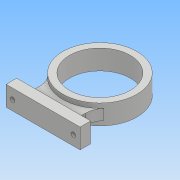
# Autodesk Inventor part: 15528 - 40mm - 1 0.25inch Universal Plastic Pipe Clip c-w Spacer Block (PP)
Saved by Autodesk Inventor 2018.1 (Build 221171000, 171)
## iProperties
Created: 2019-03-20
Part Number: 15528 - 40mm - 1 0.25inch Universal Plastic Pipe Clip c-w Spacer Block (PP)
Material: Generic
Document SubType Name: Modeling
Designer: James
Density: 1 g/cm^3
Appearance: Default
Author: James
Autodesk Inventor part; units mm, degrees
ref_plane "YZ Plane" through (0, 0, 0) normal (1, 0, 0) x (0, 1, 0)
ref_plane "XZ Plane" through (0, 0, 0) normal (0, 1, 0) x (-1, 0, 0)
ref_plane "XY Plane" through (0, 0, 0) normal (0, 0, 1) x (1, 0, 0)
sketch "Sketch1" plane through (0, 0, 0) normal (0, 0, 1) x (1, 0, 0)
  circle A0 centre (0, 0) radius 23
  circle A1 centre (0, 0) radius 28
  dimension "d0" = 46
  dimension "d1" = 56
  constraints: 2 centre point, 2 coincident
  measures "d0" diameter of A0
  measures "d1" diameter of A1
extrude "Extrusion1" add sketch "Sketch1" along normal mid plane 15
sketch "Sketch2" plane through (0, 0, 0) normal (0, 1, 0) x (-1, 0, 0)
  line L0 (17.5, -4) -> (-17.5, -4)
  line L1 (-17.5, -4) -> (-17.5, 4)
  line L2 (-17.5, 4) -> (17.5, 4)
  line L3 (17.5, 4) -> (17.5, -4)
  point P0 (0, 0)
  dimension "d4" = 8
  dimension "d5" = 4
  dimension "d6" = 35
  dimension "d7" = 17.5
  constraints: 8 end point, 2 parallel, 1 horizontal, 1 perpendicular
  measures "d4" distance of L0.end L1.end
  measures "d5" distance from line of point (0, 0) L0
  measures "d6" distance of L1.end L2.end
  measures "d7" distance from line of L3 point (0, 0)
extrude "Extrusion2" add sketch "Sketch2" against normal blind 35
sketch "Sketch3" plane through (0, -35, 0) normal (0, -1, 0) x (1, 0, 0)
  line L0 (-28, 7.5) -> (28, 7.5)
  line L1 (28, 7.5) -> (28, -7.5)
  line L2 (28, -7.5) -> (-28, -7.5)
  line L3 (-28, -7.5) -> (-28, 7.5)
  line L4 (-17.5, -4) -> (-17.5, 4) projected
  line L5 (-17.5, 4) -> (17.5, 4) projected
  line L6 (17.5, 4) -> (17.5, -4) projected
  line L7 (17.5, -4) -> (-17.5, -4) projected
  line L8 (-28, -7.5) -> (28, -7.5) projected
  line L9 (28, 7.5) -> (-28, 7.5) projected
  point P0 (0, 0)
  constraints: 8 end point, 2 parallel, 1 horizontal, 1 perpendicular
extrude "Extrusion3" add sketch "Sketch3" along normal blind 8 contours L0 L1 L2 L3 | L4 L5 L6 L7
sketch "Sketch4" plane through (0, 0, 7.5) normal (0, 0, 1) x (1, 0, 0)
  circle A0 centre (0, 0) radius 23 projected
extrude "Extrusion4" cut sketch "Sketch4" against normal through all
fillet "Fillet1" radius 15 2 edges at (-17.5, -21.8575, 0) (17.5, -21.8575, 0)
sketch "Sketch5" plane through (0, -35, 0) normal (0, 1, 0) x (1, 0, 0)
  line L0 (28, 7.5) -> (28, -7.5) projected
  line L1 (-28, -7.5) -> (-28, 7.5) projected
  point P0 (0, 0)
  point P1 (-23, 0)
  point P2 (23, 0)
  point P3 (28, 0)
  dimension "d15" = 5
  dimension "d16" = 5
  constraints: 2 horizontal alignment, 1 midpoint
  measures "d15" distance from line of point (-23, 0) L1
  measures "d16" distance from line of point (23, 0) L0
hole "Hole1" at (-23, -35, 0) at (23, -35, 0) direction (0, -1, 0) diameter 3.4 end through all counterbore diameter 6.5 counterbore depth 3 clearance for "Socket Head Cap Screw" size "M3" standard "Ansi Metric M Profile"
equation "\"d5\" = 0.5 * d4"
equation "\"d7\" = 0.5 * d6"
equation "\"d16\" = d15"
body "Solid1"
